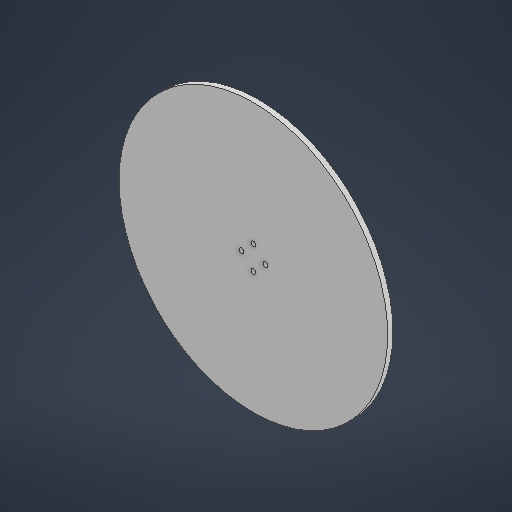
# Autodesk Inventor part: bàn xoay
Saved by Autodesk Inventor 2027.1 (Build 311270010, 270A)
## iProperties
Created: 2026-08-14
Part Number: bàn xoay
Material: Generic
Document SubType Name: Sheet Metal
Designer: MSI
Density: 1 g/cm^3
Sheet Metal Rule: Default_mm
Appearance: Default
Author: MSI
Autodesk Inventor part; units mm, degrees
ref_plane "YZ Plane" through (0, 0, 0) normal (1, 0, 0) x (0, 1, 0)
ref_plane "XZ Plane" through (0, 0, 0) normal (0, 1, 0) x (-1, 0, 0)
ref_plane "XY Plane" through (0, 0, 0) normal (0, 0, 1) x (1, 0, 0)
sketch "Sketch1" plane through (0, 0, 0) normal (0, 0, 1) x (1, 0, 0)
  circle A0 centre (0, 0) radius 90
  circle A1 centre (0, 8) radius 1.65
  circle A2 centre (-8, 0) radius 1.65
  circle A3 centre (0, -8) radius 1.65
  circle A4 centre (8, 0) radius 1.65
  dimension "d0" = 180
  dimension "d1" = 3.3
  dimension "d2" = 8
  dimension "d5" = 360
  constraints: 5 centre point, 1 coincident, 9 other
  measures "d0" diameter of A0
  measures "d1" diameter of A1
  measures "d2" distance of A1.centre point (0, 0)
extrude "Extrusion1" add sketch "Sketch1" along normal blind 3.5
equation "\"BendRadius\" = Thickness"
equation "\"BendReliefWidth\" = Thickness"
equation "\"BendReliefDepth\" = 0.5 * Thickness"
equation "\"CornerReliefSize\" = 4 * Thickness"
equation "\"MinimumRemnant\" = 2 * Thickness"
equation "\"TransitionRadius\" = BendRadius"
equation "\"JacobiRadiusSize\" = BendRadius"
equation "\"GapSize\" = Thickness"
equation "\"Thickness\" = 0.5"
body "Solid1"
